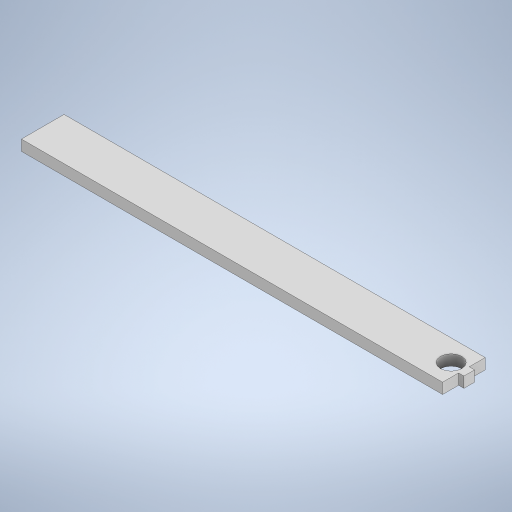
# Autodesk Inventor part: Zaxix
Saved by Autodesk Inventor 2023 (Build 270158000, 158)
## iProperties
Created: 2023-11-27
Part Number: Zaxix
Material: Generic
Document SubType Name: Modeling
Designer: Mustapha
Density: 1 g/cm^3
Appearance: Default
Author: Mustapha
Autodesk Inventor part; units mm, degrees
ref_plane "YZ Plane" through (0, 0, 0) normal (1, 0, 0) x (0, 1, 0)
ref_plane "XZ Plane" through (0, 0, 0) normal (0, 1, 0) x (-1, 0, 0)
ref_plane "XY Plane" through (0, 0, 0) normal (0, 0, 1) x (1, 0, 0)
sketch "Sketch1" plane through (0, 0, 0) normal (0, 1, 0) x (-1, 0, 0)
  line L0 (-100, 10) -> (100, 10)
  line L1 (100, 10) -> (100, -10)
  line L2 (100, -10) -> (-100, -10)
  line L3 (-100, -10) -> (-100, 10)
  line L4 (-100, 10) -> (100, -10) construction
  line L5 (100, 10) -> (-100, -10) construction
  point P0 (0, 0)
  dimension "d0" = 200
  dimension "d1" = 20
  constraints: 12 end point, 2 midpoint, 2 parallel, 1 horizontal, 1 perpendicular
  measures "d0" distance of L0.start L0.end
  measures "d1" distance between parallel lines of L2 L0
extrude "Extrusion1" add sketch "Sketch1" along normal blind 5
sketch "Sketch2" plane through (0, 5, 0) normal (0, 1, 0) x (1, 0, 0)
  line L0 (97.5, 2.5) -> (102.5, 2.5)
  line L1 (102.5, 2.5) -> (102.5, -2.5)
  line L2 (102.5, -2.5) -> (97.5, -2.5)
  line L3 (97.5, -2.5) -> (97.5, 2.5)
  line L4 (100, -10) -> (100, 10) projected
  line L5 (97.5, 2.5) -> (102.5, -2.5) construction
  line L6 (102.5, 2.5) -> (97.5, -2.5) construction
  line L7 (97.5, -2.5) -> (97.5, -10)
  line L8 (-100, -10) -> (100, -10) projected
  line L9 (97.5, -10) -> (100, -10)
  line L10 (100, -10) -> (100, 10)
  line L11 (100, 10) -> (-100, 10) projected
  line L12 (97.5, 10) -> (97.5, 2.5)
  point P0 (0, 0)
  point P1 (100, 0)
  point P2 (100, 2.5)
  point P3 (100, -2.5)
  dimension "d4" = 5
  dimension "d5" = 5
  constraints: 20 end point, 3 equal length, 3 midpoint, 3 perpendicular, 3 point on line, 1 horizontal
  measures "d4" distance between parallel lines of L2 L0
  measures "d5" distance of L1.end L2.end
extrude "Extrusion2" cut sketch "Sketch2" against normal blind 5 contours L12 L11 L4 L0 | L2 L4 L8 L7
sketch "Sketch3" plane through (0, 5, 0) normal (0, 1, 0) x (1, 0, 0)
  circle A0 centre (91.5, 0) radius 5
  line L0 (97.5, -10) -> (97.5, -2.5) projected
  point P0 (0, 0)
  dimension "d8" = 10
  dimension "d9" = 6
  constraints: 1 centre point
  measures "d8" diameter of A0
  measures "d9" distance from line of L0 A0.centre
extrude "Extrusion3" cut sketch "Sketch3" against normal blind 5
body "Solid1"
